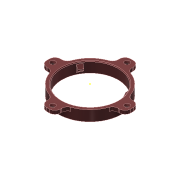
# Autodesk Inventor part: Основание бутылки
Saved by Autodesk Inventor 2022 (Build 260153000, 153)
## iProperties
Created: 2025-01-31
Part Number: Основание бутылки
Material: Типовые
Document SubType Name: Modeling
Designer: Ivan
Density: 1 g/cm^3
Appearance: Бирюзовый
Author: Ivan
Autodesk Inventor part; units mm, degrees
ref_plane "YZ Plane" through (0, 0, 0) normal (1, 0, 0) x (0, 1, 0)
ref_plane "XZ Plane" through (0, 0, 0) normal (0, 1, 0) x (-1, 0, 0)
ref_plane "XY Plane" through (0, 0, 0) normal (0, 0, 1) x (1, 0, 0)
sketch "Эскиз8" plane through (0, 0, 0) normal (1, 0, 0) x (0, 1, 0)
  line L0 (0, 0) -> (76.8443, 0) construction
  line L1 (52.5, 40) -> (48.5, 36) construction
  line L2 (48.5, 36) -> (46.5, 36) projected
  line L3 (46.5, 36) -> (42.5, 40) projected
  line L4 (52.4379, 40.15) -> (48.4379, 36.15)
  line L5 (48.4379, 36.15) -> (46.5621, 36.15)
  line L6 (46.5621, 36.15) -> (42.5621, 40.15)
  line L7 (42.5621, 40.15) -> (40, 40.15)
  line L8 (40, 40) -> (40, 0) projected
  line L9 (40, 40.15) -> (40, 45.15)
  line L10 (52.4379, 40.15) -> (55, 40.15)
  line L11 (55, 40.15) -> (55, 45.15)
  line L12 (55, 45.15) -> (40, 45.15)
  line L13 (55, 40) -> (55, -40) construction
  line L14 (55, 40) -> (40, 40) construction
  point P0 (40, 38.1462)
  dimension "d46" = 0.15
  dimension "d47" = 0.15
  dimension "d48" = 0.15
  dimension "d49" = 0.15
  dimension "d50" = 0.15
  dimension "d51" = 5
  constraints: 18 end point, 5 perpendicular, 3 horizontal, 3 parallel, 2 collinear
  measures "d46" distance between parallel lines of L1 L4
  measures "d47" distance between parallel lines of L2 L5
  measures "d48" distance between parallel lines of L3 L6
  measures "d49" distance between parallel lines of L14 L10
  measures "d50" distance between parallel lines of L14 L7
  measures "d51" distance of L10.end L11.end
revolve "Вращение3" add sketch "Эскиз8" angle 10 mid plane about axis through (0, 0, 0) along (0, 1, 0)
pattern_circular "Круговой массив2" count 3 over 360 about axis through (0, -10, 0) along (0, 1, 0) of "Вращение3"
sketch "Эскиз9" plane through (3.9351, 40, 44.9782) normal (0.9961947, 0, -0.0871557) x (-0.0871557, 0, -0.9961947)
  line L0 (0, 15) -> (0, 0) projected
  line L1 (0, 0) -> (5, 0) projected
  line L2 (5, 0) -> (5, 2.5621) projected
  line L3 (5, 2.5621) -> (9, 6.5621) construction
  line L4 (9, 6.5621) -> (9, 8.4379) projected
  line L5 (9, 8.4379) -> (5, 12.4379) construction
  line L6 (5, 12.4379) -> (5, 15) projected
  line L7 (5, 15) -> (0, 15) projected
  line L8 (9, 8.4379) -> (5, 12.4379) projected
  line L9 (5, 12.4379) -> (5, 2.5621)
  line L10 (5.15, 15) -> (5.15, 0) construction
  line L11 (45.15, -52.6066) -> (45.15, 35.6396) projected
  point P0 (45.15, -40)
  constraints: 2 end point, 1 parallel
revolve "Вращение4" add sketch "Эскиз9" angle 360 about axis through (0, -10, 0) along (0, 1, 0)
sketch "Эскиз10" plane through (0, 55, 0) normal (0, 1, 0) x (1, 0, 0)
  circle A0 centre (0, 0) radius 45.15 construction
  line L0 (0, 0) -> (-70.0694, 0) construction
  line L1 (-40.15, -10) -> (-60, -10)
  line L2 (-60, -10) -> (-60, 10)
  line L3 (-60, 10) -> (-40.15, 10)
  line L4 (-40.15, 10) -> (-40.15, -10)
  line L5 (-40.15, -10) -> (-60, 10) construction
  line L6 (-60, -10) -> (-40.15, 10) construction
  circle A1 centre (-53.075, 0) radius 1.7
  circle A2 centre (0, -53.075) radius 1.7
  line L7 (10, -60) -> (-10, -60)
  line L8 (10, -40.15) -> (10, -60)
  line L9 (-10, -40.15) -> (10, -40.15)
  line L10 (-10, -60) -> (-10, -40.15)
  circle A3 centre (53.075, 0) radius 1.7
  line L11 (60, 10) -> (60, -10)
  line L12 (40.15, 10) -> (60, 10)
  line L13 (40.15, -10) -> (40.15, 10)
  line L14 (60, -10) -> (40.15, -10)
  circle A4 centre (0, 53.075) radius 1.7
  line L15 (-10, 60) -> (10, 60)
  line L16 (-10, 40.15) -> (-10, 60)
  line L17 (10, 40.15) -> (-10, 40.15)
  line L18 (10, 60) -> (10, 40.15)
  circle A5 centre (0, 0) radius 40.15 projected
  point P0 (0, 0)
  point P1 (-50.075, 0)
  dimension "d58" = 20
  dimension "d60" = 60
  dimension "d61" = 3.4
  dimension "d62" = 3
  dimension "d65" = 360
  constraints: 38 end point, 4 centre point, 2 horizontal, 2 midpoint, 2 parallel, 2 point on line, 1 horizontal alignment, 1 perpendicular, 1 tangent, 41 other
  measures "d58" distance of L1.end L2.end
  measures "d60" distance from line of point (0, 0) L2
  measures "d61" diameter of A1
  measures "d62" distance of point (-50.075, 0) A1.centre
extrude "Выдавливание3" add sketch "Эскиз10" against normal blind 5 contours L17 L16 L15 L18 | L13 L12 L11 L14 | L9 L8 L7 L10 | L1 L2 L3 L4
fillet "Сопряжение1" radius 8 16 edges at (10, 52.5, -44.0287) (-10, 52.5, -44.0287) (10, 52.5, -60) (-10, 52.5, -60) (-44.0287, 52.5, -10) (-60, 52.5, -10) (-60, 52.5, 10) (-44.0287, 52.5, 10) (-10, 52.5, 44.0287) (10, 52.5, 44.0287) (10, 52.5, 60) (-10, 52.5, 60) (44.0287, 52.5, 10) (44.0287, 52.5, -10) (60, 52.5, -10) (60, 52.5, 10)
chamfer "Фаска4" distance 2 angle 45 4 edges at (-1.7, 55, 53.075) (-54.775, 55, 0) (51.375, 55, 0) (-1.7, 55, -53.075)
chamfer "Фаска9" distance 1 angle 45 10 edges at (-29.6017, 55, 27.1249) (29.6017, 55, 27.1249) (-1.7513, 55, 40.1118) (1.7513, 55, 40.1118) (-39.1983, 55, -8.6901) (39.1983, 55, -8.6901) (-34.7709, 55, -20.075) (34.7709, 55, -20.075) (-18.5392, 55, -35.6135) (18.5392, 55, -35.6135)
sketch "Эскиз19" plane through (-2, 55, -60) normal (0, 1, 0) x (1, 0, 0)
  point P0 (2, -60)
equation "\"d47\" = d46"
equation "\"d48\" = d47"
equation "\"d49\" = d46"
equation "\"d50\" = d46"
